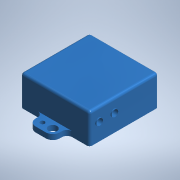
# Autodesk Inventor part: IMU
Saved by Autodesk Inventor 2022.1 (Build 261234000, 234)
## iProperties
Part Number: IMU
Material: Genérico
Document SubType Name: Modelado
Designer: seb_0
Appearance: Cian
Author: seb_0
Autodesk Inventor part; units mm, degrees
ref_plane "Plano YZ" through (0, 0, 0) normal (1, 0, 0) x (0, 1, 0)
ref_plane "Plano XZ" through (0, 0, 0) normal (0, 1, 0) x (-1, 0, 0)
ref_plane "Plano XY" through (0, 0, 0) normal (0, 0, 1) x (1, 0, 0)
sketch "Boceto1" plane through (0, 0, 0) normal (0, 1, 0) x (-1, 0, 0)
  line L0 (0, 0) -> (25.4, 0)
  line L1 (25.4, 0) -> (25.4, -25.4)
  line L2 (25.4, -25.4) -> (0, -25.4)
  line L3 (0, -25.4) -> (0, 0)
  dimension "d0" = 25.4
  dimension "d1" = 25.4
  constraints: 8 end point, 2 parallel, 1 horizontal, 1 perpendicular
  measures "d0" distance of L0.end L1.end
  measures "d1" distance of L1.end L2.end
extrude "Extrusión1" add sketch "Boceto1" along normal blind 11.176
sketch "Boceto2" plane through (0, 0, 0) normal (0, -1, 0) x (1, 0, 0)
  line L0 (-17.145, 0) -> (-17.145, 5.2578)
  line L1 (-17.145, 5.2578) -> (-8.255, 5.2578)
  line L2 (-8.255, 5.2578) -> (-8.255, 0)
  line L3 (-25.4, 0) -> (0, 0) projected
  line L4 (0, -25.4) -> (-25.4, -25.4) projected
  line L5 (-8.255, -25.4) -> (-8.255, -30.6578)
  line L6 (-8.255, -30.6578) -> (-17.145, -30.6578)
  line L7 (-25.4, -25.4) -> (-25.4, 0) projected
  line L8 (-25.4, -12.7) -> (0, -12.7)
  line L9 (0, 0) -> (0, -25.4) projected
  circle A0 centre (-10.795, 2.7178) radius 1.5875
  circle A1 centre (-10.795, -28.1178) radius 1.5875
  circle A2 centre (-14.605, 2.7178) radius 0.8001
  circle A3 centre (-14.605, -28.1178) radius 0.8001
  line L10 (-10.795, 2.7178) -> (-10.795, -28.1178)
  line L11 (-14.605, 2.7178) -> (-14.605, -28.1178)
  line L12 (-17.145, -30.6578) -> (-17.145, -25.4)
  circle A4 centre (-10.795, 2.7178) radius 2.54
  circle A5 centre (-10.795, -28.1178) radius 2.54
  circle A6 centre (-14.605, 2.7178) radius 2.54
  circle A7 centre (-14.605, -28.1178) radius 2.54
  circle A8 centre (-19.05, 1.905) radius 1.905
  line L13 (-25.4, 0) -> (0, 0) projected
  circle A9 centre (-6.35, 1.905) radius 1.905
  circle A10 centre (-6.35, -27.305) radius 1.905
  circle A11 centre (-19.05, -27.305) radius 1.905
  point P0 (-9.175, -12.7)
  point P1 (-10.795, -12.7)
  point P2 (-14.605, -12.7)
  point P3 (-12.7, -12.7)
  point P4 (-10.795, -30.6578)
  point P5 (-8.255, -28.1178)
  point P6 (-8.255, -27.305)
  point P7 (-6.35, -25.4)
  point P8 (-19.05, -25.4)
  point P9 (-17.145, -27.305)
  point P10 (-17.145, -28.1178)
  point P11 (-14.605, -30.6578)
  point P12 (-14.605, 5.2578)
  point P13 (-17.145, 2.7178)
  point P14 (-17.145, 1.905)
  point P15 (-19.05, 0)
  point P16 (-6.35, 0)
  point P17 (-8.255, 1.905)
  point P18 (-8.255, 2.7178)
  point P19 (-10.795, 5.2578)
  dimension "d4" = 5.2578
  dimension "d5" = 5.2578
  dimension "d6" = 3.175
  dimension "d7" = 3.175
  dimension "d8" = 1.6002
  dimension "d9" = 1.6002
  dimension "d12" = 30.8356
  dimension "d13" = 1.905
  dimension "d14" = 1.905
  dimension "d15" = 3.81
  dimension "d16" = 3.81
  dimension "d17" = 3.81
  dimension "d18" = 3.81
  constraints: 18 end point, 15 tangent, 12 centre point, 6 point on line, 5 midpoint, 5 vertical, 3 perpendicular, 2 parallel
  measures "d4" distance of L1.end L2.end
  measures "d5" distance of L5.start L5.end
  measures "d6" diameter of A0
  measures "d7" diameter of A1
  measures "d8" diameter of A2
  measures "d9" diameter of A3
  measures "d12" distance of L10.start L10.end
  measures "d13" distance from line of point (-12.7, -12.7) L10
  measures "d14" distance from line of point (-12.7, -12.7) L11
  measures "d15" diameter of A8
  measures "d16" diameter of A9
  measures "d17" diameter of A10
  measures "d18" diameter of A11
extrude "Extrusión2" add sketch "Boceto2" against normal blind 1.905 contours L3 A8 L0 | L0 A6 L11 L3 | L11 A6 A4 L10 L3 | A6 A4 | L10 A4 L2 L3 | L1 A4 A6 | L2 A9 L3 | A4 A6 A0 L10 | L10 A0 A6 A4 | A4 A6 A0 | L11 A7 L12 L4 | L4 L10 A5 A7 L11 | L4 L5 A5 L10 | L12 A11 L4 | A7 A5 | L4 A10 L5 | A5 A7 A1 L10 | L10 A1 A7 A5 | A7 A1 A5 | A5 L6 A7
sketch "Boceto3" plane through (0, 0, 0) normal (1, 0, 0) x (0, 0, -1)
  line L0 (25.4, 11.176) -> (0, 11.176) projected
  line L1 (12.7, 11.176) -> (12.7, 0)
  line L2 (25.4, 0) -> (0, 0) projected
  circle A0 centre (3.4036, 6.477) radius 1.2065
  circle A1 centre (8.9916, 6.477) radius 1.2065
  dimension "d23" = 3.7084
  dimension "d24" = 9.2964
  dimension "d25" = 6.477
  dimension "d26" = 6.477
  dimension "d27" = 2.413
  constraints: 2 centre point, 2 end point, 2 midpoint, 1 equal radius
  measures "d23" distance from line of L1 A1.centre
  measures "d24" distance from line of L1 A0.centre
  measures "d25" distance from line of L2 A0.centre
  measures "d26" distance from line of L2 A1.centre
  measures "d27" diameter of A0
fillet "Empalme1" radius 0.9525 4 edges at (-12.7, 11.176, 0) (-12.7, 11.176, -25.4) (-25.4, 11.176, -12.7) (0, 11.176, -12.7)
fillet "Empalme2" radius 0.9525 8 edges at (-0.279, 10.897, -0.279) (0, 5.1117, 0) (-25.121, 10.897, -0.279) (-25.4, 5.1117, 0) (-0.279, 10.897, -25.121) (0, 5.1117, -25.4) (-25.121, 10.897, -25.121) (-25.4, 5.1117, -25.4)
extrude "Extrusión3" cut sketch "Boceto3" against normal blind 2.6924
sketch "Boceto4" plane through (0, 0, -0.9525) normal (1, 0, 0) x (0, 0, -1)
  circle A0 centre (2.4511, 6.477) radius 1.2065 projected
  circle A1 centre (8.0391, 6.477) radius 1.2065 projected
  circle A2 centre (8.0391, 6.477) radius 1.27
  circle A3 centre (2.4511, 6.477) radius 1.27
  point P0 (-0.9525, 0)
  dimension "d30" = 2.54
  constraints: 2 centre point, 2 coincident, 1 equal radius
  measures "d30" diameter of A2
extrude "Extrusión4" add sketch "Boceto4" along normal blind 0.3556
